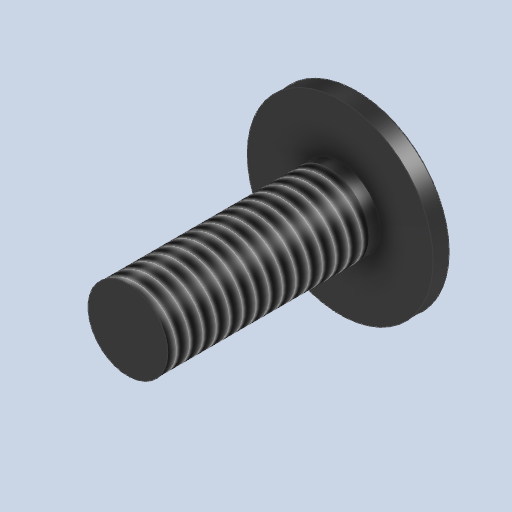
# Autodesk Inventor part: 620103008
Saved by Autodesk Inventor 2022 (Build 260153000, 153)
## iProperties
Part Number: 620103008
Material: ステンレス鋼 AISI 304
Document SubType Name: Modeling
Designer: Masato Kubotera
Density: 6.25777 g/cm^3
Appearance: 光沢 - 黒
Catalog Web Link: https://jp.misumi-ec.com/vona2/detail/221000862966/?HissuCode=620103008
Description: ReadyMade
Mass: 0.578947 g
Surface Area: 1.79669 cm^2
Volume: 0.0925166 cm^3
Author: Masato Kubotera
Comments: Width across flats : 2
Autodesk Inventor part; units mm, degrees
ref_plane "YZ Plane" through (0, 0, 0) normal (1, 0, 0) x (0, 1, 0)
ref_plane "XZ Plane" through (0, 0, 0) normal (0, 1, 0) x (-1, 0, 0)
ref_plane "XY Plane" through (0, 0, 0) normal (0, 0, 1) x (1, 0, 0)
sketch "スケッチ1" plane through (0, 0, 0) normal (0, 1, 0) x (-1, 0, 0)
  line L0 (0, 0) -> (-1.1547, 0)
  line L1 (-2.6, 1.05) -> (-3.5, 1.05)
  line L2 (-3.5, 1.05) -> (-3.5, 1.65)
  line L3 (-3.5, 1.65) -> (-1.5, 1.65)
  line L4 (-1.5, 1.65) -> (-1.5, 9.65)
  line L5 (-1.5, 9.65) -> (0, 9.65)
  line L6 (0, 9.65) -> (0, 0)
  arc A0 (-2.6, 1.05) -> (-1.1547, 0) centre (-1.1547, 1.5197) ccw
  dimension "d0" = 5.2
  dimension "d1" = 7
  dimension "d3" = 1.65
  dimension "d4" = 0.6
  dimension "d5" = 2.3094
  dimension "d6" = 8
  dimension "d7" = 3
  constraints: 14 end point, 6 perpendicular, 2 point on circle, 1 centre point, 1 horizontal, 1 tangent
  measures "d0" diameter of L1.start L6
  measures "d1" diameter of L1.end L6
  measures "d3" vertical distance of L0.end L2.end
  measures "d4" distance of L1.end L2.end
  measures "d5" diameter of L0.end L6
  measures "d6" distance of L3.end L4.end
  measures "d7" diameter of L4.end L6
revolve "回転1" add sketch "スケッチ1" angle 360 about axis through (0, 0, 9.65) along (0, 0, -1)
thread "ねじ1" size "M3x0.5" class "6g" standard "ANSI Metric M Profile" length 7.57
sketch "スケッチ2" plane through (0, 0, 0) normal (0, 0, -1) x (-1, 0, 0)
  circle A0 centre (0, 0) radius 1.1547 projected
  line L0 (0, 1.1547) -> (1, 0.5774)
  line L1 (1, 0.5774) -> (1, -0.5774)
  line L2 (1, -0.5774) -> (0, -1.1547)
  line L3 (0, -1.1547) -> (-1, -0.5774)
  line L4 (-1, -0.5774) -> (-1, 0.5774)
  line L5 (-1, 0.5774) -> (0, 1.1547)
  point P0 (0, 0)
  constraints: 12 end point, 1 coincident, 1 vertical, 1 vertical alignment, 14 other
extrude "押し出し1" cut sketch "スケッチ2" against normal blind 1.05 contours L1 L2 L3 L4 L5 L0
